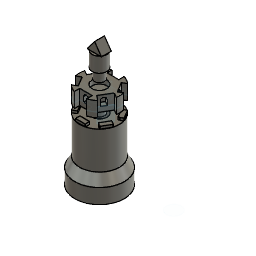
rook (Autodesk Fusion 360 design; units mm, degrees)
part number: 2026-07-03-02-51-02-908
Autodesk Fusion 360 part; units mm, degrees
note: some values were not read from the file. Set by a fixed rule: which sketch regions a step uses.
sketch "Sketch1" plane through (0, 0, 0) normal (0, 0, 1) x (1, 0, 0)
  line L0 (12.7, 0) -> (12.7, 7.62)
  line L1 (12.7, 7.62) -> (10.16, 12.7)
  line L2 (10.16, 12.7) -> (10.16, 31.75)
  line L3 (10.16, 31.75) -> (0, 31.75)
  line L4 (0, 31.75) -> (0, 0)
  line L5 (0, 0) -> (12.7, 0)
  dimension "d1" = 19.05
  constraint vertical L0
  constraint parallel L0 L2
  constraint perpendicular L2 L3
  constraint coincident L4.end L5.start
  constraint perpendicular L3 L4
  constraint perpendicular L0 L5
  measures "d1" distance of L1.end L2.end
revolve "Revolve1" add sketch "Sketch1" angle 360 about axis through (0, 31.75, 0) along (0, -1, 0) makes body 1
sketch "Sketch2" plane through (0, 31.75, 0) normal (0, 1, 0) x (-1, 0, 0)
  circle A0 centre (0, 0) radius 10.16
  circle A1 centre (0, 0) radius 12.7
  line L0 (2.5391, 9.8376) -> (-2.54, 9.8376)
  line L1 (-2.54, 9.8376) -> (-2.54, 8.3136)
  line L2 (-2.54, 8.3136) -> (2.5391, 8.3136)
  line L3 (2.5391, 8.3136) -> (2.5391, 9.8376)
  dimension "d3" = 1.524
  constraint horizontal L0
  constraint vertical L1
  constraint horizontal L2
  constraint vertical L3
  constraint coincident A0 L0.start
  measures "d3" distance of L0.start L2.end
sketch "Sketch3" plane through (0, 31.75, 0) normal (0, 1, 0) x (-1, 0, 0)
  circle A0 centre (0, 0) radius 10.16
  line L0 (2.3981, 9.8729) -> (-2.54, 9.8729)
  line L1 (-2.54, 9.8729) -> (-2.54, 7.5869)
  line L2 (-2.54, 7.5869) -> (2.3981, 7.5869)
  line L3 (2.3981, 7.5869) -> (2.3981, 9.8729)
  dimension "d6" = 2.286
  constraint horizontal L0
  constraint vertical L1
  constraint horizontal L2
  constraint vertical L3
  constraint coincident A0 L0.start
  measures "d6" distance of L0.start L2.end
extrude "Extrude2" add sketch "Sketch3" along normal blind 1.27 contours A0 L0 L1 L2 L3 bodies 1
extrude "Extrude1" add sketch "Sketch2" along normal blind 1.27 contours L0 L1 L2 L3 bodies 1
pattern_circular "C-Pattern1" count 6 over 360 about axis through (0, 31.75, 0) along (0, -1, 0) of bodies 1 makes body 2 at (-7.0168, 33.02, 5.0288) makes body 3 at (-7.8635, 33.02, -3.5623) makes body 4 at (-0.8467, 33.02, -8.5912) makes body 5 at (7.0168, 33.02, -5.0288) makes body 6 at (7.8635, 33.02, 3.5623)
ref_plane "WorkPlane1" through (0, 32.385, 17.4929) normal (0, 0, 1) x (1, 0, 0)
sketch "Sketch5" plane through (0, 0, 0) normal (0, 0, 1) x (1, 0, 0)
ref_plane "WorkPlane2" through (0.1396, 36.83, 0.081) normal (0, 1, 0) x (-0.866025, 0, -0.5)
sketch "Sketch6" plane through (0, 36.83, 0) normal (0, 1, 0) x (1, 0, 0)
  circle A0 centre (0, 0) radius 10.2035
  line L0 (-3.3059, -9.6531) -> (-3.3059, -6.8526)
  line L1 (-3.3059, -6.8526) -> (3.0674, -6.8526)
  line L2 (3.0674, -6.8526) -> (3.0674, -9.7315)
  line L3 (6.7422, -7.6586) -> (4.2421, -5.6126)
  line L4 (4.2421, -5.6126) -> (7.62, 0)
  line L5 (7.62, 0) -> (10.0942, -1.4891)
  line L6 (9.9136, 2.4149) -> (7.874, 1.27)
  line L7 (7.874, 1.27) -> (4.826, 6.35)
  line L8 (4.826, 6.35) -> (6.8486, 7.5636)
  line L9 (-3.1955, 9.6902) -> (-3.1955, 7.112)
  line L10 (-3.1955, 7.112) -> (2.794, 7.112)
  line L11 (2.794, 7.112) -> (2.794, 9.8135)
  line L12 (-7.0708, 7.3563) -> (-4.826, 6.096)
  line L13 (-4.826, 6.096) -> (-7.6512, 1.064)
  line L14 (-7.6512, 1.064) -> (-9.9306, 2.3438)
  line L15 (-9.9199, -2.3888) -> (-7.7227, -1.1487)
  line L16 (-7.7227, -1.1487) -> (-4.826, -6.096)
  line L17 (-4.826, -6.096) -> (-7.0357, -7.3898)
  constraint coincident A0.centre origin
  constraint coincident A0 L0.start
  constraint vertical L0
  constraint perpendicular L0 L1
  constraint coincident A0 L2.end
  constraint perpendicular L1 L2
  constraint coincident A0 L3.start
  constraint coincident A0 L5.end
  constraint perpendicular L4 L5
  constraint coincident A0 L6.start
  constraint coincident A0 L8.end
  constraint perpendicular L7 L8
  constraint coincident A0 L9.start
  constraint vertical L9
  constraint perpendicular L9 L10
  constraint coincident A0 L11.end
  constraint perpendicular L10 L11
  constraint coincident A0 L12.start
  constraint perpendicular L12 L13
  constraint coincident A0 L14.end
  constraint perpendicular L13 L14
  constraint coincident A0 L15.start
  constraint coincident A0 L17.end
  constraint perpendicular L16 L17
extrude "Extrude3" add sketch "Sketch6" along normal blind 7.62 separate body contours A0 L0 L1 L2 L3 L4 L5 L6 L7 L8 L9 L10 L11 L12 L13 L14 L15 L16 L17 makes body 7
move_body "Move1" bodies 7 to x (1, 0, 0) y (0, 1, 0) z (0, 0, 1) at (0, -5.08, 0)
sketch "Sketch7" plane through (0, 0, 6.8526) normal (0, 0, 1) x (1, 0, 0)
  line L0 (-3.3059, 31.75) -> (3.0674, 31.75)
  line L1 (3.0674, 31.75) -> (3.0674, 39.37)
  line L2 (3.0674, 39.37) -> (-3.3059, 39.37)
  line L3 (-3.3059, 39.37) -> (-3.3059, 31.75)
  line L4 (-1.27, 34.29) -> (1.27, 34.29)
  line L5 (1.27, 34.29) -> (1.27, 36.83)
  line L6 (-1.27, 34.29) -> (-1.27, 36.83)
  arc A0 (1.27, 36.83) -> (-1.27, 36.83) centre (0, 36.83) ccw
  constraint horizontal L4
  constraint perpendicular L4 L5
  constraint perpendicular L4 L6
  constraint tangent L5 A0
  constraint tangent L6 A0
extrude "Extrude4" cut sketch "Sketch7" against normal blind 2.54 contours L4 L5 L6 A0 bodies 7
sketch "Sketch8" plane through (5.5939, 0, 3.3666) normal (0.856797, 0, 0.515654) x (0.515654, 0, -0.856797)
  line L0 (-2.6214, 31.75) -> (3.9293, 31.75)
  line L1 (3.9293, 31.75) -> (3.9293, 39.37)
  line L2 (3.9293, 39.37) -> (-2.6214, 39.37)
  line L3 (-2.6214, 39.37) -> (-2.6214, 31.75)
sketch "Sketch9" plane through (5.5939, 0, 3.3666) normal (0.856797, 0, 0.515654) x (0.515654, 0, -0.856797)
  line L0 (-1.27, 34.29) -> (-1.27, 36.83)
  line L1 (-1.27, 36.83) -> (-1.27, 34.29)
  line L2 (1.27, 34.29) -> (1.27, 36.83)
  arc A0 (1.27, 36.83) -> (-1.27, 36.83) centre (0, 36.83) ccw
  line L3 (1.27, 34.29) -> (-1.27, 34.29)
  constraint vertical L0
  constraint parallel L0 L2
  constraint tangent L2 A0
  constraint tangent L1 A0
  constraint perpendicular L1 L3
extrude "Extrude5" cut sketch "Sketch9" against normal blind 2.54 bodies 7
sketch "Sketch10" plane through (6.35, 0, -3.81) normal (0.857493, 0, -0.514496) x (-0.514496, 0, -0.857493)
  line L0 (-2.9621, 31.75) -> (2.9621, 31.75)
  line L1 (2.9621, 31.75) -> (2.9621, 39.37)
  line L2 (2.9621, 39.37) -> (-2.9621, 39.37)
  line L3 (-2.9621, 39.37) -> (-2.9621, 31.75)
  line L4 (-1.27, 34.29) -> (-1.27, 36.83)
  line L5 (1.27, 34.29) -> (-1.27, 34.29)
  line L6 (1.27, 34.29) -> (1.27, 36.83)
  arc A0 (1.27, 36.83) -> (-1.27, 36.83) centre (0, 36.83) ccw
  constraint vertical L4
  constraint perpendicular L4 L5
  constraint perpendicular L5 L6
  constraint tangent L6 A0
  constraint tangent L4 A0
sketch "Sketch11" plane through (-3.1955, 0, 0) normal (1, 0, 0) x (0, 0, -1)
  line L0 (7.112, 31.75) -> (9.6902, 31.75)
  line L1 (9.6902, 31.75) -> (9.6902, 39.37)
  line L2 (9.6902, 39.37) -> (7.112, 39.37)
  line L3 (7.112, 39.37) -> (7.112, 31.75)
sketch "Sketch12" plane through (0, 0, -7.112) normal (0, 0, -1) x (-1, 0, 0)
  line L0 (-2.794, 31.75) -> (3.1955, 31.75)
  line L1 (3.1955, 31.75) -> (3.1955, 39.37)
  line L2 (3.1955, 39.37) -> (-2.794, 39.37)
  line L3 (-2.794, 39.37) -> (-2.794, 31.75)
  line L4 (-1.27, 34.29) -> (1.27, 34.29)
  line L5 (1.27, 34.29) -> (1.27, 36.83)
  line L6 (-1.27, 34.29) -> (-1.27, 36.83)
  arc A0 (1.27, 36.83) -> (-1.27, 36.83) centre (0, 36.83) ccw
  constraint horizontal L4
  constraint perpendicular L4 L5
  constraint perpendicular L4 L6
  constraint tangent L5 A0
  constraint tangent L6 A0
sketch "Sketch13" plane through (-6.2716, 0, -3.5212) normal (-0.871967, 0, -0.489565) x (-0.489565, 0, 0.871967)
  line L0 (-2.9529, 31.75) -> (2.818, 31.75)
  line L1 (2.818, 31.75) -> (2.818, 39.37)
  line L2 (2.818, 39.37) -> (-2.9529, 39.37)
  line L3 (-2.9529, 39.37) -> (-2.9529, 31.75)
  line L4 (-1.27, 34.29) -> (1.27, 34.29)
  line L5 (1.27, 34.29) -> (1.27, 36.83)
  line L6 (-1.27, 34.29) -> (-1.27, 36.83)
  arc A0 (1.27, 36.83) -> (-1.27, 36.83) centre (0, 36.83) ccw
  constraint horizontal L4
  constraint perpendicular L4 L5
  constraint perpendicular L4 L6
  constraint tangent L5 A0
  constraint tangent L6 A0
sketch "Sketch14" plane through (-6.252, 0, 3.6606) normal (-0.862959, 0, 0.505275) x (0.505275, 0, 0.862959)
  line L0 (-2.9108, 31.75) -> (2.8221, 31.75)
  line L1 (2.8221, 31.75) -> (2.8221, 39.37)
  line L2 (2.8221, 39.37) -> (-2.9108, 39.37)
  line L3 (-2.9108, 39.37) -> (-2.9108, 31.75)
  line L4 (-1.27, 34.29) -> (1.27, 34.29)
  line L5 (1.27, 34.29) -> (1.27, 36.83)
  line L6 (-1.27, 34.29) -> (-1.27, 36.83)
  arc A0 (1.27, 36.83) -> (-1.27, 36.83) centre (0, 36.83) ccw
  constraint parallel L0 L4
  constraint perpendicular L4 L5
  constraint perpendicular L4 L6
  constraint tangent L5 A0
  constraint tangent L6 A0
extrude "Extrude6" cut sketch "Sketch10" against normal blind 2.54 contours L4 L5 L6 A0 bodies 7
extrude "Extrude7" cut sketch "Sketch12" against normal blind 2.54 contours L4 L5 L6 A0 bodies 7
extrude "Extrude8" cut sketch "Sketch13" against normal blind 2.54 contours L4 L5 L6 A0 bodies 7
extrude "Extrude9" cut sketch "Sketch14" against normal blind 2.54 contours L4 L5 L6 A0 bodies 7
move_body "Move2" bodies 7 to x (1, 0, 0) y (0, 1, 0) z (0, 0, 1) at (22.86, 0, 0)
sketch "Sketch15" plane through (0, 31.75, 0) normal (0, 1, 0) x (-1, 0, 0)
  line L0 (7.2501, -7.1177) -> (5.9302, -6.3557)
  line L1 (5.9302, -6.3557) -> (6.0008, -6.2336)
  line L2 (6.0008, -6.2336) -> (5.3714, -5.8703)
  line L3 (5.3714, -5.8703) -> (7.8405, -1.5938)
  line L4 (7.8405, -1.5938) -> (9.7894, -2.719)
  arc A0 (9.7894, -2.719) -> (7.2501, -7.1177) centre (0, 0) ccw
  circle A1 centre (0, 0) radius 3.81
  dimension "d27" = 7.62
  constraint concentric A0 A1
  measures "d27" diameter of A1
extrude "Extrude10" cut sketch "Sketch15" against normal blind 5.08 contours A1 bodies 1 2 3 4 5 6
sketch "Sketch16" plane through (0, 31.75, 0) normal (0, -1, 0) x (1, 0, 0)
  arc A0 (15.7892, -7.3563) -> (19.6645, -9.6902) centre (22.86, 0) ccw
  line L0 (19.6645, -9.6902) -> (19.6645, -7.112)
  line L1 (19.6645, -7.112) -> (25.654, -7.112)
  line L2 (25.654, -7.112) -> (25.654, -9.8135)
  arc A1 (25.654, -9.8135) -> (29.7086, -7.5636) centre (22.86, 0) ccw
  line L3 (29.7086, -7.5636) -> (27.686, -6.35)
  line L4 (27.686, -6.35) -> (30.734, -1.27)
  line L5 (30.734, -1.27) -> (32.7736, -2.4149)
  arc A2 (32.7736, -2.4149) -> (32.9542, 1.4891) centre (22.86, 0) ccw
  line L6 (32.9542, 1.4891) -> (30.48, 0)
  line L7 (30.48, 0) -> (27.1021, 5.6126)
  line L8 (27.1021, 5.6126) -> (29.6022, 7.6586)
  arc A3 (29.6022, 7.6586) -> (25.9274, 9.7315) centre (22.86, 0) ccw
  line L9 (25.9274, 9.7315) -> (25.9274, 6.8526)
  line L10 (25.9274, 6.8526) -> (19.5541, 6.8526)
  line L11 (19.5541, 6.8526) -> (19.5541, 9.6531)
  arc A4 (19.5541, 9.6531) -> (15.8243, 7.3898) centre (22.86, 0) ccw
  line L12 (15.8243, 7.3898) -> (18.034, 6.096)
  line L13 (18.034, 6.096) -> (15.1373, 1.1487)
  line L14 (15.1373, 1.1487) -> (12.9401, 2.3888)
  arc A5 (12.9401, 2.3888) -> (12.9294, -2.3438) centre (22.86, 0) ccw
  line L15 (12.9294, -2.3438) -> (15.2088, -1.064)
  line L16 (15.2088, -1.064) -> (18.034, -6.096)
  line L17 (18.034, -6.096) -> (15.7892, -7.3563)
  circle A6 centre (22.86, 0) radius 2.54
  dimension "d30" = 5.08
  constraint concentric A0 A6
  measures "d30" diameter of A6
extrude "Extrude11" add sketch "Sketch16" along normal blind 5.08 contours A6 bodies 7
move_body "Move3" bodies 7 to x (1, 0, 0) y (0, 1, 0) z (0, 0, 1) at (-22.86, 0, 0)
sketch "Sketch17" plane through (0, 39.37, 0) normal (0, 1, 0) x (-1, 0, 0)
  arc A0 (3.1955, -9.6902) -> (7.0708, -7.3563) centre (0, 0) ccw
  line L0 (7.0708, -7.3563) -> (4.826, -6.096)
  line L1 (4.826, -6.096) -> (7.6512, -1.064)
  line L2 (7.6512, -1.064) -> (9.9306, -2.3438)
  arc A1 (9.9306, -2.3438) -> (9.9199, 2.3888) centre (0, 0) ccw
  line L3 (9.9199, 2.3888) -> (7.7227, 1.1487)
  line L4 (7.7227, 1.1487) -> (4.826, 6.096)
  line L5 (4.826, 6.096) -> (7.0357, 7.3898)
  arc A2 (7.0357, 7.3898) -> (3.3059, 9.6531) centre (0, 0) ccw
  line L6 (3.3059, 9.6531) -> (3.3059, 6.8526)
  line L7 (3.3059, 6.8526) -> (-3.0674, 6.8526)
  line L8 (-3.0674, 6.8526) -> (-3.0674, 9.7315)
  arc A3 (-3.0674, 9.7315) -> (-6.7422, 7.6586) centre (0, 0) ccw
  line L9 (-6.7422, 7.6586) -> (-4.2421, 5.6126)
  line L10 (-4.2421, 5.6126) -> (-7.62, 0)
  line L11 (-7.62, 0) -> (-10.0942, 1.4891)
  arc A4 (-10.0942, 1.4891) -> (-9.9136, -2.4149) centre (0, 0) ccw
  line L12 (-9.9136, -2.4149) -> (-7.874, -1.27)
  line L13 (-7.874, -1.27) -> (-4.826, -6.35)
  line L14 (-4.826, -6.35) -> (-6.8486, -7.5636)
  arc A5 (-6.8486, -7.5636) -> (-2.794, -9.8135) centre (0, 0) ccw
  line L15 (-2.794, -9.8135) -> (-2.794, -7.112)
  line L16 (-2.794, -7.112) -> (3.1955, -7.112)
  line L17 (3.1955, -7.112) -> (3.1955, -9.6902)
sketch "Sketch18" plane through (0, 0, 0) normal (0, 1, 0) x (1, 0, 0)
  circle A0 centre (38.1, 0) radius 3.81
  dimension "d33" = 7.62
  measures "d33" diameter of A0
extrude "Extrude12" add sketch "Sketch18" along normal blind 7.62 separate body makes body 8
sketch "Sketch19" plane through (0, 39.37, 0) normal (0, 1, 0) x (-1, 0, 0)
  circle A0 centre (0, 0) radius 3.81
  dimension "d36" = 7.62
  constraint coincident A0.centre origin
  measures "d36" diameter of A0
extrude "Extrude13" cut sketch "Sketch19" against normal blind 2.54 bodies 7
sketch "Sketch26" plane through (0, 0, 0) normal (0, 1, 0) x (1, 0, 0)
  circle A0 centre (38.1, 0) radius 2.54
  dimension "d53" = 5.08
  measures "d53" diameter of A0
extrude "Extrude19" add sketch "Sketch26" against normal blind 5.08 bodies 8
sketch "Sketch27" plane through (0, 7.62, 0) normal (0, 1, 0) x (-1, 0, 0)
  circle A0 centre (-38.1, 0) radius 3.81
sketch "Sketch28" plane through (0, 0, 0) normal (0, 0, 1) x (1, 0, 0)
  line L0 (34.29, 7.62) -> (38.1, 12.7)
  line L1 (38.1, 12.7) -> (41.6316, 7.62)
  line L2 (41.6316, 7.62) -> (34.29, 7.62)
  constraint horizontal L2
extrude "Extrude20" add sketch "Sketch28" along normal blind 2.54 bodies 8
extrude "Extrude21" add 1 faces at (38.0072, 9.3133, 0) along direction (0, 0, -1) blind 2.54 on bodies 8 bodies 8
move_body "Move16" bodies 8 to x (1, 0, 0) y (0, 1, 0) z (0, 0, 1) at (-38.1, 39.37, 0)
sketch "Sketch29" plane through (0, 0, 0) normal (0, 0, 1) x (1, 0, 0)
move_body "Move17" bodies 7 to x (1, 0, 0) y (0, 1, 0) z (0, 0, 1) at (0, 5.08, 0)
move_body "Move18" bodies 8 to x (1, 0, 0) y (0, 1, 0) z (0, 0, 1) at (0, 12.7, 0)
combine "Combine2" operation add target body 1 tool bodies 5 3 6 2 4
extrude "Extrude14" [suppressed]
sketch "Sketch20" plane through (0, 10.16, 0) normal (0, 1, 0) x (-1, 0, 0)
  circle A0 centre (-38.1, 0) radius 3.81
  line L0 (-40.64, 2.54) -> (-35.56, 2.54)
  line L1 (-35.56, 2.54) -> (-35.56, -2.54)
  line L2 (-35.56, -2.54) -> (-40.64, -2.54)
  line L3 (-40.64, -2.54) -> (-40.64, 2.54)
  line L4 (-40.64, 2.54) -> (-35.56, -2.54) construction
  line L5 (-35.56, 2.54) -> (-40.64, -2.54) construction
  point P0 (-38.1, 0)
  constraint horizontal L0
  constraint perpendicular L0 L1
  constraint parallel L0 L2
  constraint parallel L1 L3
  constraint coincident L4 P0
  constraint coincident L5 P0
  constraint coincident P0 A0.centre
extrude "Extrude15" [suppressed]
sketch "Sketch21" plane through (0, 16.51, 0) normal (0, 1, 0) x (-1, 0, 0)
  line L0 (-40.64, -2.54) -> (-35.56, -2.54)
  line L1 (-35.56, -2.54) -> (-35.56, 2.54)
  line L2 (-35.56, 2.54) -> (-40.64, 2.54)
  line L3 (-40.64, 2.54) -> (-40.64, -2.54)
sketch "Sketch22" plane through (0, 0, 0) normal (0, 0, 1) x (1, 0, 0)
  line L0 (35.56, 16.51) -> (38.1, 19.05)
  line L1 (40.64, 16.51) -> (38.1, 19.05)
  line L2 (35.56, 16.51) -> (40.64, 16.51)
  constraint perpendicular L0 L1
  constraint horizontal L2
extrude "Extrude16" [suppressed]
extrude "Extrude17" [suppressed]
move_body "Move4" [suppressed]
move_body "Move5" [suppressed]
sketch "Sketch23" plane through (0, 0, 2.54) normal (0, 0, 1) x (1, 0, 0)
  line L0 (-2.6729, 41.9299) -> (2.4071, 41.9299)
  line L1 (2.4071, 41.9299) -> (2.4071, 48.2799)
  line L2 (2.4071, 48.2799) -> (-0.1329, 50.8199)
  line L3 (-0.1329, 50.8199) -> (-2.6729, 48.2799)
  line L4 (-2.6729, 48.2799) -> (-2.6729, 41.9299)
hole "Hole1" [suppressed]
sketch "Sketch24" plane through (0, 0, 0) normal (1, 0, 0) x (0, 0, -1)
  circle A0 centre (0, 22.86) radius 2.54
  dimension "d50" = 5.08
  measures "d50" diameter of A0
extrude "Extrude18" [suppressed]
move_body "Move6" [suppressed]
move_body "Move7" [suppressed]
move_body "Move8" [suppressed]
move_body "Move9" [suppressed]
sketch "Sketch25" plane through (0, 0, 0) normal (0, 0, 1) x (1, 0, 0)
  circle A0 centre (0, 0) radius 5.08
  constraint coincident A0.centre origin
move_body "Move10" [suppressed]
move_body "Move11" [suppressed]
combine "Combine1" [suppressed]
move_body "Move12" [suppressed]
move_body "Move13" [suppressed]
move_body "Move14" [suppressed]
move_body "Move15" [suppressed]
sketch "Sketch4" plane through (0, 0, 17.4929) normal (0, 0, 1) x (1, 0, 0)
  line L0 (-1.27, 33.02) -> (-1.27, 34.29)
  line L1 (-1.27, 34.29) -> (0, 34.29)
  line L2 (0, 34.29) -> (0, 33.02)
  line L3 (0, 33.02) -> (1.27, 33.02)
  line L4 (1.27, 33.02) -> (1.27, 34.29)
  line L5 (1.27, 34.29) -> (2.2539, 34.29)
  line L6 (2.2539, 34.29) -> (2.2539, 33.02)
  line L7 (2.2539, 33.02) -> (1.27, 33.02)
  line L8 (0, 33.02) -> (-1.27, 33.02)
  constraint vertical L0
  constraint perpendicular L0 L1
  constraint perpendicular L1 L2
  constraint perpendicular L2 L3
  constraint perpendicular L3 L4
  constraint perpendicular L4 L5
  constraint perpendicular L5 L6
  constraint perpendicular L4 L7
  constraint perpendicular L0 L8
named bodies: "main"
